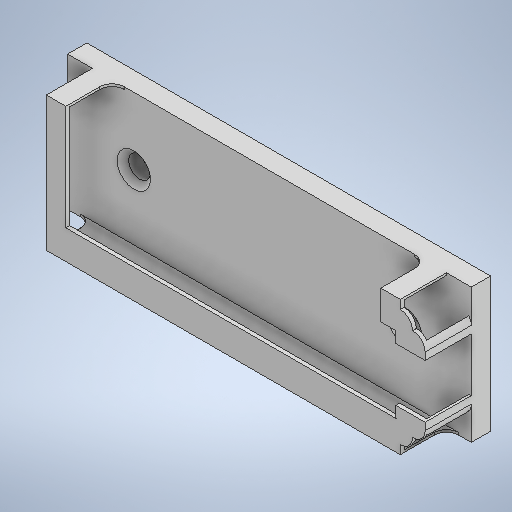
# Autodesk Inventor part: USB_HUB_MOUNT
Saved by Autodesk Inventor 2025 (Build 290162010, 162A)
## iProperties
Created: 2024-10-18
Part Number: USB_HUB_MOUNT
Material: Generic
Document SubType Name: Modeling
Designer: shubh
Density: 1 g/cm^3
Appearance: Default
Author: shubh
Autodesk Inventor part; units mm, degrees
ref_plane "YZ Plane" through (0, 0, 0) normal (1, 0, 0) x (0, 1, 0)
ref_plane "XZ Plane" through (0, 0, 0) normal (0, 1, 0) x (-1, 0, 0)
ref_plane "XY Plane" through (0, 0, 0) normal (0, 0, 1) x (1, 0, 0)
sketch "Sketch1" plane through (0, 0, 0) normal (0, 0, 1) x (1, 0, 0)
  line L0 (52.5, -17.5) -> (-52.5, -17.5)
  line L1 (-52.5, -17.5) -> (-52.5, 17.5)
  line L2 (-52.5, 17.5) -> (52.5, 17.5)
  line L3 (52.5, 17.5) -> (52.5, -17.5)
  line L4 (52.5, -17.5) -> (-52.5, 17.5) construction
  line L5 (-52.5, -17.5) -> (52.5, 17.5) construction
  point P0 (0, 0)
  dimension "d0" = 105
  dimension "d1" = 35
  constraints: 12 end point, 2 midpoint, 2 parallel, 1 horizontal, 1 perpendicular
  measures "d0" distance of L1.end L2.end
  measures "d1" distance of L0.end L1.end
extrude "Extrusion1" add sketch "Sketch1" along normal blind 5
sketch "Sketch2" plane through (0, 0, 5) normal (0, 0, 1) x (1, 0, 0)
  line L0 (52.5, 17.5) -> (-52.5, 17.5) construction
  line L1 (43.5, 17.5) -> (43.5, -17.5) construction
  line L2 (-52.5, -17.5) -> (52.5, -17.5) construction
  line L3 (52.5, -17.5) -> (52.5, 17.5) construction
  line L4 (-43.5, 17.5) -> (-43.5, -17.5) construction
  line L5 (-52.5, 17.5) -> (-52.5, -17.5) construction
  line L6 (-46.0403, 16.8926) -> (-40.9597, 16.8926)
  line L7 (-40.9597, 16.8926) -> (-40.9597, 17.5)
  line L8 (-40.9597, 17.5) -> (-46.0403, 17.5)
  line L9 (-46.0403, 17.5) -> (-46.0403, 16.8926)
  line L10 (-46.0403, 16.8926) -> (-40.9597, 17.5) construction
  line L11 (-40.9597, 16.8926) -> (-46.0403, 17.5) construction
  line L12 (0, 17.5) -> (0, -17.5) construction
  line L13 (-52.5, 0) -> (52.5, 0) construction
  line L14 (-52.5, 17.5) -> (52.5, 17.5) construction
  line L15 (40.9597, 16.8926) -> (40.9597, 17.5)
  line L16 (40.9597, 17.5) -> (46.0403, 17.5)
  line L17 (46.0403, 17.5) -> (46.0403, 16.8926)
  line L18 (46.0403, 16.8926) -> (40.9597, 17.5) construction
  line L19 (40.9597, 16.8926) -> (46.0403, 16.8926)
  line L20 (52.5, -17.5) -> (-52.5, -17.5) construction
  line L21 (-46.0403, -16.8926) -> (-40.9597, -16.8926)
  line L22 (-40.9597, -17.5) -> (-46.0403, -17.5)
  line L23 (-46.0403, -17.5) -> (-46.0403, -16.8926)
  line L24 (46.0403, -17.5) -> (46.0403, -16.8926)
  line L25 (-52.5, -17.5) -> (52.5, -17.5) construction
  line L26 (40.9597, -17.5) -> (46.0403, -17.5)
  line L27 (40.9597, -16.8926) -> (46.0403, -16.8926)
  line L28 (-40.9597, -16.8926) -> (40.9597, -16.8926)
  line L29 (40.9597, -17.5) -> (-40.9597, -17.5)
  line L30 (52.5, 9.5) -> (-52.5, 9.5) construction
  line L31 (52.5, -9.5) -> (-52.5, -9.5) construction
  line L32 (52.5, 6.96) -> (51.8904, 6.96)
  line L33 (51.8904, 6.96) -> (51.8904, 12.04)
  line L34 (51.8904, 12.04) -> (52.5, 12.04)
  line L35 (52.5, 12.04) -> (52.5, 6.96)
  line L36 (52.5, 6.96) -> (51.8904, 12.04) construction
  line L37 (51.8904, 6.96) -> (52.5, 12.04) construction
  line L38 (52.5, -6.96) -> (51.8904, -6.96)
  line L39 (51.8904, -6.96) -> (51.8904, -12.04)
  line L40 (51.8904, -12.04) -> (52.5, -12.04)
  line L41 (52.5, -12.04) -> (52.5, -6.96)
  point P0 (0, 0)
  point P1 (-43.5, 17.1963)
  point P2 (52.1952, 9.5)
  dimension "d4" = 9
  dimension "d5" = 9
  dimension "d6" = 8
  dimension "d7" = 8
  dimension "d8" = 0.6096
  dimension "d9" = 5.08
  constraints: 76 end point, 22 symmetric about line, 14 point on line, 8 midpoint, 5 perpendicular, 4 horizontal, 4 parallel, 3 collinear, 1 vertical
  measures "d4" distance between parallel lines of L3 L1
  measures "d5" distance between parallel lines of L5 L4
  measures "d6" distance between parallel lines of L0 L30
  measures "d7" distance between parallel lines of L2 L31
  measures "d8" distance of L33.end L34.end
  measures "d9" distance of L34.end L32.start
extrude "Extrusion2" add sketch "Sketch2" along normal blind 12
sketch "Sketch3" plane through (0, 0, 5) normal (0, 0, 1) x (1, 0, 0)
  line L0 (52.5, -17.5) -> (52.5, 17.5) construction
  line L1 (52.5, 0) -> (-52.5, 0) construction
  line L2 (-52.5, 17.5) -> (-52.5, -17.5) construction
  line L3 (0, -17.697) -> (0, 17.5) construction
  line L4 (40.9597, 17.5) -> (-40.9597, 17.5) construction
  line L5 (-46.0403, 17.5) -> (-52.5, 17.5) construction
  line L6 (52.5, -17.697) -> (-52.5, 17.5) construction
  line L7 (52.5, 17.5) -> (46.0403, 17.5) construction
  line L8 (-52.5, -17.5) -> (52.5, 17.5) construction
  circle A0 centre (35.2834, 0) radius 2.85
  circle A1 centre (-35.2834, 0) radius 2.85
  point P0 (0, 0)
  dimension "d12" = 5.7
  constraints: 8 end point, 3 midpoint, 2 centre point, 1 point on line, 1 symmetric about line, 1 other
  measures "d12" diameter of A0
extrude "Extrusion3" cut sketch "Sketch3" against normal blind 12
chamfer "Chamfer1" distance 1.5 angle 45 2 edges at (32.4334, 0, 5) (-38.1334, 0, 5)
sketch "Sketch4" plane through (-46.0403, -16.8926, 5) normal (0, 1, 0) x (1, 0, 0)
  line L0 (0, 0) -> (92.0806, 0) projected
  line L1 (0, 0) -> (0, -12) projected
  line L2 (92.0806, -12) -> (0, -12) projected
  line L3 (92.0806, 0) -> (92.0806, -12) projected
  line L4 (97.9307, 0) -> (97.9307, -12) projected
  line L5 (97.9307, 0) -> (97.9307, -12) projected
  line L6 (92.0806, 0) -> (92.0806, -12) projected
  line L7 (0, 0) -> (0, -12) projected
  line L8 (92.0806, -12) -> (0, -12)
  line L9 (0, -12) -> (0, -11)
  line L10 (0, -11) -> (92.0806, -11)
  line L11 (92.0806, -11) -> (92.0806, -12)
  point P0 (46.0403, 5)
  dimension "d18" = 1
  constraints: 8 end point, 2 parallel, 1 horizontal, 1 perpendicular, 1 point on line
  measures "d18" distance of L8.end L9.end
extrude "Extrusion4" add sketch "Sketch4" along normal blind 7 contours L10 L3 L2 L1
sketch "Sketch5" plane through (51.8904, 6.96, 5) normal (-1, 0, 0) x (0, 0, 1)
  line L0 (12, 5.08) -> (12, 0) projected
  line L1 (0, 0) -> (12, 0) projected
  line L2 (12, 5.08) -> (11, 5.08)
  line L3 (11, 5.08) -> (11, 0)
  line L4 (11, 0) -> (12, 0)
  line L5 (12, 0) -> (12, 5.08)
  line L6 (0, -13.92) -> (12, -13.92) projected
  line L7 (0, -19) -> (12, -19) projected
  line L8 (12, -13.92) -> (11, -13.92)
  line L9 (11, -13.92) -> (11, -19)
  line L10 (11, -19) -> (12, -19)
  line L11 (12, -19) -> (12, -13.92)
  point P0 (-5, -6.96)
  dimension "d21" = 1
  dimension "d22" = 1
  constraints: 16 end point, 4 parallel, 2 horizontal, 2 perpendicular, 2 point on line
  measures "d21" distance of L4.end L3.end
  measures "d22" distance of L10.end L9.end
extrude "Extrusion5" add sketch "Sketch5" along normal blind 7
fillet "Fillet1" radius 3.175 1 edges at (46.0403, -12.04, 16.5) inverted yes
fillet "Fillet2" radius 3.175 1 edges at (52.5, -12.04, 11)
fillet "Fillet3" radius 3.175 1 edges at (52.5, 12.04, 11)
sketch "Sketch7" plane through (40.9597, 16.8926, 5) normal (0, -1, 0) x (1, 0, 0)
  line L0 (0, 0) -> (0, 12) projected
  line L1 (5.0806, 0) -> (5.0806, 12) projected
  line L2 (0, 12) -> (5.0806, 12)
  line L3 (5.0806, 12) -> (5.0806, 11)
  line L4 (5.0806, 11) -> (0, 11)
  line L5 (0, 11) -> (0, 12)
  point P0 (-40.9597, -5)
  dimension "d32" = 1
  constraints: 8 end point, 2 parallel, 1 horizontal, 1 perpendicular, 1 point on line
  measures "d32" distance of L2.end L3.end
extrude "Extrusion7" add sketch "Sketch7" along normal blind 7
fillet "Fillet4" radius 3.175 1 edges at (46.0403, 12.04, 16.5) inverted yes
sketch "Sketch8" plane through (-46.0403, 16.8926, 5) normal (0, -1, 0) x (1, 0, 0)
  line L0 (5.0806, 12) -> (0, 12) projected
  line L1 (5.0806, 0) -> (5.0806, 12) projected
  line L2 (0, 12) -> (5.0806, 12)
  line L3 (5.0806, 12) -> (5.0806, 11)
  line L4 (5.0806, 11) -> (0, 11)
  line L5 (0, 11) -> (0, 12)
  point P0 (46.0403, -5)
  dimension "d36" = 1
  constraints: 8 end point, 2 parallel, 1 horizontal, 1 perpendicular, 1 point on line
  measures "d36" distance of L2.end L3.end
extrude "Extrusion8" add sketch "Sketch8" along normal blind 27.6375
fillet "Fillet5" radius 3.175 2 edges at (40.9597, 17.1963, 5) (-40.9597, 17.1963, 5)
fillet "Fillet6" radius 3.175 2 edges at (-46.0403, -17.1963, 5) (46.0403, -17.1963, 5)
body "Solid1"
